Autodesk Fusion 360 part; units mm, degrees
(part 5 of 5)
  spline S33 degree 5 poles (-94.5307, 28.5823) (-94.5425, 28.575) (-94.566, 28.5604) (-94.6013, 28.5385) (-94.6482, 28.509) (-94.7065, 28.4721) (-94.7647, 28.4349) (-94.8226, 28.3975) (-94.8803, 28.3599) (-94.9377, 28.322) (-94.9949, 28.284) (-95.0518, 28.2458) (-95.1085, 28.2073) (-95.165, 28.1687) (-95.2212, 28.1298) (-95.2771, 28.0907) (-95.3328, 28.0514) (-95.3883, 28.0119) (-95.4435, 27.9721) (-95.4984, 27.9322) (-95.5531, 27.892) (-95.6074, 27.8517) (-95.6616, 27.8111) (-95.7154, 27.7703) (-95.769, 27.7293) (-95.8223, 27.688) (-95.8753, 27.6466) (-95.9281, 27.6049) (-95.9805, 27.563) (-96.0327, 27.5208) (-96.0845, 27.4785) (-96.1361, 27.4359) (-96.1874, 27.3931) (-96.2383, 27.3501) (-96.289, 27.3069) (-96.3393, 27.2634) (-96.3894, 27.2197) (-96.4391, 27.1758) (-96.4885, 27.1316) (-96.5375, 27.0872) (-96.5863, 27.0426) (-96.6346, 26.9977) (-96.6827, 26.9526) (-96.7303, 26.9073) (-96.7777, 26.8617) (-96.8246, 26.8158) (-96.8712, 26.7698) (-96.9175, 26.7234) (-96.9633, 26.6769) (-97.0088, 26.6301) (-97.0539, 26.583) (-97.0985, 26.5356) (-97.1427, 26.488) (-97.1865, 26.44) (-97.2298, 26.3918) (-97.2726, 26.3434) (-97.3151, 26.2946) (-97.3572, 26.2457) (-97.3988, 26.1965) (-97.44, 26.1469) (-97.4805, 26.0971) (-97.5204, 26.0468) (-97.5595, 25.9961) (-97.5979, 25.9449) (-97.6356, 25.8934) (-97.6728, 25.8417) (-97.7097, 25.7897) (-97.7462, 25.7375) (-97.7822, 25.6851) (-97.8172, 25.6321) (-97.8506, 25.5783) (-97.8756, 25.5344) (-97.8932, 25.5007) (-97.9043, 25.478) (-97.9097, 25.4666) knots -1 -1 -1 -1 -1 -1 -0.98571429 -0.97142857 -0.95714286 -0.94285714 -0.92857143 -0.91428571 -0.9 -0.88571429 -0.87142857 -0.85714286 -0.84285714 -0.82857143 -0.81428571 -0.8 -0.78571429 -0.77142857 -0.75714286 -0.74285714 -0.72857143 -0.71428571 -0.7 -0.68571429 -0.67142857 -0.65714286 -0.64285714 -0.62857143 -0.61428571 -0.6 -0.58571429 -0.57142857 -0.55714286 -0.54285714 -0.52857143 -0.51428571 -0.5 -0.48571429 -0.47142857 -0.45714286 -0.44285714 -0.42857143 -0.41428571 -0.4 -0.38571429 -0.37142857 -0.35714286 -0.34285714 -0.32857143 -0.31428571 -0.3 -0.28571429 -0.27142857 -0.25714286 -0.24285714 -0.22857143 -0.21428571 -0.2 -0.18571429 -0.17142857 -0.15714286 -0.14285714 -0.12857143 -0.11428571 -0.1 -0.08571429 -0.07142857 -0.05714286 -0.04285714 -0.02857143 -0.01428571 0 0 0 0 0 0
  line L33 (-97.9097, 25.4666) -> (-97.9531, 25.3753)
  arc A67 (-99.2529, 24.8861) -> (-97.9531, 25.3753) centre (-98.8565, 25.8041) ccw
  arc A68 (-99.2529, 24.8861) -> (-100.0022, 25.1964) centre (-110, 0) ccw
  arc A69 (-100.5754, 26.4615) -> (-100.0022, 25.1964) centre (-99.6334, 26.1259) ccw
  line L34 (-100.5754, 26.4615) -> (-100.5415, 26.5567)
  spline S34 degree 5 poles (-100.5415, 26.5567) (-100.5373, 26.5686) (-100.5291, 26.5926) (-100.5177, 26.6288) (-100.5043, 26.6775) (-100.4899, 26.7392) (-100.4772, 26.8014) (-100.4656, 26.8639) (-100.4545, 26.9266) (-100.4438, 26.9894) (-100.4335, 27.0524) (-100.4238, 27.1155) (-100.4148, 27.1788) (-100.4066, 27.2423) (-100.3992, 27.306) (-100.3926, 27.37) (-100.3867, 27.4341) (-100.3813, 27.4983) (-100.3765, 27.5627) (-100.372, 27.6272) (-100.3681, 27.6918) (-100.3646, 27.7565) (-100.3616, 27.8213) (-100.3592, 27.8862) (-100.3573, 27.9513) (-100.3559, 28.0164) (-100.3549, 28.0817) (-100.3544, 28.1471) (-100.3544, 28.2125) (-100.3547, 28.2781) (-100.3555, 28.3437) (-100.3568, 28.4094) (-100.3584, 28.4752) (-100.3605, 28.541) (-100.3629, 28.607) (-100.3658, 28.673) (-100.3691, 28.739) (-100.3728, 28.8052) (-100.3769, 28.8714) (-100.3814, 28.9377) (-100.3863, 29.004) (-100.3915, 29.0704) (-100.3971, 29.1369) (-100.4031, 29.2034) (-100.4095, 29.27) (-100.4162, 29.3366) (-100.4233, 29.4032) (-100.4308, 29.47) (-100.4386, 29.5367) (-100.4468, 29.6035) (-100.4553, 29.6704) (-100.4642, 29.7373) (-100.4734, 29.8042) (-100.483, 29.8712) (-100.4929, 29.9382) (-100.5031, 30.0052) (-100.5137, 30.0723) (-100.5247, 30.1394) (-100.5359, 30.2066) (-100.5475, 30.2738) (-100.5594, 30.341) (-100.5717, 30.4082) (-100.5843, 30.4755) (-100.5972, 30.5427) (-100.6104, 30.61) (-100.624, 30.6774) (-100.6378, 30.7447) (-100.652, 30.8121) (-100.6665, 30.8795) (-100.6813, 30.9469) (-100.6964, 31.0143) (-100.7088, 31.0683) (-100.7182, 31.1088) (-100.7245, 31.1357) (-100.7277, 31.1492) knots 0 0 0 0 0 0 0.01428571 0.02857143 0.04285714 0.05714286 0.07142857 0.08571429 0.1 0.11428571 0.12857143 0.14285714 0.15714286 0.17142857 0.18571429 0.2 0.21428571 0.22857143 0.24285714 0.25714286 0.27142857 0.28571429 0.3 0.31428571 0.32857143 0.34285714 0.35714286 0.37142857 0.38571429 0.4 0.41428571 0.42857143 0.44285714 0.45714286 0.47142857 0.48571429 0.5 0.51428571 0.52857143 0.54285714 0.55714286 0.57142857 0.58571429 0.6 0.61428571 0.62857143 0.64285714 0.65714286 0.67142857 0.68571429 0.7 0.71428571 0.72857143 0.74285714 0.75714286 0.77142857 0.78571429 0.8 0.81428571 0.82857143 0.84285714 0.85714286 0.87142857 0.88571429 0.9 0.91428571 0.92857143 0.94285714 0.95714286 0.97142857 0.98571429 1 1 1 1 1 1
  arc A70 (-100.7277, 31.1492) -> (-102.4554, 31.6122) centre (-110, 0) ccw
  spline S35 degree 5 poles (-102.4554, 31.6122) (-102.4649, 31.6021) (-102.4839, 31.5819) (-102.5123, 31.5515) (-102.55, 31.511) (-102.5968, 31.4601) (-102.6433, 31.4092) (-102.6896, 31.3581) (-102.7355, 31.3068) (-102.7812, 31.2554) (-102.8266, 31.2039) (-102.8717, 31.1522) (-102.9165, 31.1004) (-102.9611, 31.0484) (-103.0053, 30.9963) (-103.0492, 30.9441) (-103.0928, 30.8917) (-103.1362, 30.8392) (-103.1792, 30.7865) (-103.2219, 30.7337) (-103.2643, 30.6808) (-103.3064, 30.6277) (-103.3482, 30.5745) (-103.3896, 30.5212) (-103.4308, 30.4677) (-103.4716, 30.414) (-103.5121, 30.3603) (-103.5522, 30.3063) (-103.592, 30.2523) (-103.6315, 30.1981) (-103.6707, 30.1438) (-103.7094, 30.0893) (-103.7479, 30.0347) (-103.786, 29.98) (-103.8237, 29.9251) (-103.8611, 29.8701) (-103.8981, 29.8149) (-103.9348, 29.7596) (-103.971, 29.7042) (-104.0069, 29.6486) (-104.0425, 29.5929) (-104.0776, 29.537) (-104.1123, 29.481) (-104.1466, 29.4249) (-104.1805, 29.3686) (-104.214, 29.3121) (-104.2471, 29.2556) (-104.2798, 29.1989) (-104.312, 29.142) (-104.3439, 29.085) (-104.3752, 29.0279) (-104.4061, 28.9706) (-104.4364, 28.9131) (-104.4663, 28.8555) (-104.4956, 28.7977) (-104.5245, 28.7398) (-104.5529, 28.6818) (-104.5809, 28.6236) (-104.6083, 28.5653) (-104.6353, 28.5068) (-104.6615, 28.4481) (-104.687, 28.3892) (-104.7117, 28.3301) (-104.7355, 28.2708) (-104.7586, 28.2113) (-104.7812, 28.1516) (-104.8033, 28.0919) (-104.8251, 28.0321) (-104.8463, 27.9721) (-104.8664, 27.9119) (-104.8848, 27.8513) (-104.8975, 27.8023) (-104.9058, 27.7653) (-104.9107, 27.7405) (-104.9129, 27.728) knots -1 -1 -1 -1 -1 -1 -0.98571429 -0.97142857 -0.95714286 -0.94285714 -0.92857143 -0.91428571 -0.9 -0.88571429 -0.87142857 -0.85714286 -0.84285714 -0.82857143 -0.81428571 -0.8 -0.78571429 -0.77142857 -0.75714286 -0.74285714 -0.72857143 -0.71428571 -0.7 -0.68571429 -0.67142857 -0.65714286 -0.64285714 -0.62857143 -0.61428571 -0.6 -0.58571429 -0.57142857 -0.55714286 -0.54285714 -0.52857143 -0.51428571 -0.5 -0.48571429 -0.47142857 -0.45714286 -0.44285714 -0.42857143 -0.41428571 -0.4 -0.38571429 -0.37142857 -0.35714286 -0.34285714 -0.32857143 -0.31428571 -0.3 -0.28571429 -0.27142857 -0.25714286 -0.24285714 -0.22857143 -0.21428571 -0.2 -0.18571429 -0.17142857 -0.15714286 -0.14285714 -0.12857143 -0.11428571 -0.1 -0.08571429 -0.07142857 -0.05714286 -0.04285714 -0.02857143 -0.01428571 0 0 0 0 0 0
  line L35 (-104.9129, 27.728) -> (-104.9312, 27.6286)
  arc A71 (-106.0601, 26.8197) -> (-104.9312, 27.6286) centre (-105.9148, 27.809) ccw
  arc A72 (-106.0601, 26.8197) -> (-106.8642, 26.9255) centre (-110, 0) ccw
  arc A73 (-107.7453, 27.9991) -> (-106.8642, 26.9255) centre (-106.7485, 27.9188) ccw
  line L36 (-107.7453, 27.9991) -> (-107.7372, 28.0998)
  spline S36 degree 5 poles (-107.7372, 28.0998) (-107.7362, 28.1124) (-107.7345, 28.1377) (-107.7328, 28.1756) (-107.7325, 28.2262) (-107.7345, 28.2895) (-107.7384, 28.3528) (-107.7433, 28.4162) (-107.7489, 28.4797) (-107.7548, 28.5431) (-107.7612, 28.6066) (-107.7681, 28.67) (-107.7758, 28.7335) (-107.7843, 28.797) (-107.7937, 28.8605) (-107.8038, 28.9239) (-107.8147, 28.9874) (-107.8262, 29.0508) (-107.8381, 29.1143) (-107.8505, 29.1777) (-107.8634, 29.2411) (-107.8768, 29.3045) (-107.8907, 29.3679) (-107.9052, 29.4312) (-107.9202, 29.4946) (-107.9357, 29.5579) (-107.9516, 29.6212) (-107.9681, 29.6844) (-107.985, 29.7477) (-108.0023, 29.8109) (-108.02, 29.8741) (-108.0382, 29.9372) (-108.0568, 30.0003) (-108.0759, 30.0634) (-108.0953, 30.1264) (-108.1152, 30.1895) (-108.1355, 30.2524) (-108.1562, 30.3154) (-108.1773, 30.3783) (-108.1988, 30.4411) (-108.2206, 30.504) (-108.2429, 30.5667) (-108.2655, 30.6295) (-108.2885, 30.6922) (-108.3119, 30.7548) (-108.3356, 30.8174) (-108.3598, 30.88) (-108.3842, 30.9425) (-108.4091, 31.005) (-108.4342, 31.0674) (-108.4598, 31.1297) (-108.4857, 31.1921) (-108.5119, 31.2543) (-108.5385, 31.3165) (-108.5654, 31.3787) (-108.5927, 31.4408) (-108.6203, 31.5029) (-108.6482, 31.5649) (-108.6764, 31.6268) (-108.705, 31.6887) (-108.7339, 31.7505) (-108.7632, 31.8123) (-108.7927, 31.874) (-108.8226, 31.9356) (-108.8528, 31.9972) (-108.8833, 32.0588) (-108.9142, 32.1202) (-108.9453, 32.1816) (-108.9767, 32.243) (-109.0085, 32.3043) (-109.0406, 32.3655) (-109.0664, 32.4144) (-109.086, 32.4511) (-109.0991, 32.4755) (-109.1057, 32.4877) knots 0 0 0 0 0 0 0.01428571 0.02857143 0.04285714 0.05714286 0.07142857 0.08571429 0.1 0.11428571 0.12857143 0.14285714 0.15714286 0.17142857 0.18571429 0.2 0.21428571 0.22857143 0.24285714 0.25714286 0.27142857 0.28571429 0.3 0.31428571 0.32857143 0.34285714 0.35714286 0.37142857 0.38571429 0.4 0.41428571 0.42857143 0.44285714 0.45714286 0.47142857 0.48571429 0.5 0.51428571 0.52857143 0.54285714 0.55714286 0.57142857 0.58571429 0.6 0.61428571 0.62857143 0.64285714 0.65714286 0.67142857 0.68571429 0.7 0.71428571 0.72857143 0.74285714 0.75714286 0.77142857 0.78571429 0.8 0.81428571 0.82857143 0.84285714 0.85714286 0.87142857 0.88571429 0.9 0.91428571 0.92857143 0.94285714 0.95714286 0.97142857 0.98571429 1 1 1 1 1 1
  arc A74 (-109.1057, 32.4877) -> (-110.8943, 32.4877) centre (-110, 0) ccw
  spline S37 degree 5 poles (-110.8943, 32.4877) (-110.9009, 32.4755) (-110.914, 32.4511) (-110.9336, 32.4144) (-110.9594, 32.3655) (-110.9915, 32.3043) (-111.0233, 32.243) (-111.0547, 32.1816) (-111.0858, 32.1202) (-111.1167, 32.0588) (-111.1472, 31.9972) (-111.1774, 31.9356) (-111.2073, 31.874) (-111.2368, 31.8123) (-111.2661, 31.7505) (-111.295, 31.6887) (-111.3236, 31.6268) (-111.3518, 31.5649) (-111.3797, 31.5029) (-111.4073, 31.4408) (-111.4346, 31.3787) (-111.4615, 31.3165) (-111.4881, 31.2543) (-111.5143, 31.1921) (-111.5402, 31.1297) (-111.5658, 31.0674) (-111.5909, 31.005) (-111.6158, 30.9425) (-111.6402, 30.88) (-111.6644, 30.8174) (-111.6881, 30.7548) (-111.7115, 30.6922) (-111.7345, 30.6295) (-111.7571, 30.5667) (-111.7794, 30.504) (-111.8012, 30.4411) (-111.8227, 30.3783) (-111.8438, 30.3154) (-111.8645, 30.2524) (-111.8848, 30.1895) (-111.9047, 30.1264) (-111.9241, 30.0634) (-111.9432, 30.0003) (-111.9618, 29.9372) (-111.98, 29.8741) (-111.9977, 29.8109) (-112.015, 29.7477) (-112.0319, 29.6844) (-112.0484, 29.6212) (-112.0643, 29.5579) (-112.0798, 29.4946) (-112.0948, 29.4312) (-112.1093, 29.3679) (-112.1232, 29.3045) (-112.1366, 29.2411) (-112.1495, 29.1777) (-112.1619, 29.1143) (-112.1738, 29.0508) (-112.1853, 28.9874) (-112.1962, 28.9239) (-112.2063, 28.8605) (-112.2157, 28.797) (-112.2242, 28.7335) (-112.2319, 28.67) (-112.2388, 28.6066) (-112.2452, 28.5431) (-112.2511, 28.4797) (-112.2567, 28.4162) (-112.2616, 28.3528) (-112.2655, 28.2895) (-112.2675, 28.2262) (-112.2672, 28.1756) (-112.2655, 28.1377) (-112.2638, 28.1124) (-112.2628, 28.0998) knots -1 -1 -1 -1 -1 -1 -0.98571429 -0.97142857 -0.95714286 -0.94285714 -0.92857143 -0.91428571 -0.9 -0.88571429 -0.87142857 -0.85714286 -0.84285714 -0.82857143 -0.81428571 -0.8 -0.78571429 -0.77142857 -0.75714286 -0.74285714 -0.72857143 -0.71428571 -0.7 -0.68571429 -0.67142857 -0.65714286 -0.64285714 -0.62857143 -0.61428571 -0.6 -0.58571429 -0.57142857 -0.55714286 -0.54285714 -0.52857143 -0.51428571 -0.5 -0.48571429 -0.47142857 -0.45714286 -0.44285714 -0.42857143 -0.41428571 -0.4 -0.38571429 -0.37142857 -0.35714286 -0.34285714 -0.32857143 -0.31428571 -0.3 -0.28571429 -0.27142857 -0.25714286 -0.24285714 -0.22857143 -0.21428571 -0.2 -0.18571429 -0.17142857 -0.15714286 -0.14285714 -0.12857143 -0.11428571 -0.1 -0.08571429 -0.07142857 -0.05714286 -0.04285714 -0.02857143 -0.01428571 0 0 0 0 0 0
  line L37 (-112.2628, 28.0998) -> (-112.2547, 27.9991)
  arc A75 (-113.1358, 26.9255) -> (-112.2547, 27.9991) centre (-113.2515, 27.9188) ccw
  arc A76 (-113.1358, 26.9255) -> (-113.9399, 26.8197) centre (-110, 0) ccw
  arc A77 (-115.0688, 27.6286) -> (-113.9399, 26.8197) centre (-114.0852, 27.809) ccw
  line L38 (-115.0688, 27.6286) -> (-115.0871, 27.728)
  spline S38 degree 5 poles (-115.0871, 27.728) (-115.0893, 27.7405) (-115.0942, 27.7653) (-115.1025, 27.8023) (-115.1152, 27.8513) (-115.1336, 27.9119) (-115.1537, 27.9721) (-115.1749, 28.0321) (-115.1967, 28.0919) (-115.2188, 28.1516) (-115.2414, 28.2113) (-115.2645, 28.2708) (-115.2883, 28.3301) (-115.313, 28.3892) (-115.3385, 28.4481) (-115.3647, 28.5068) (-115.3917, 28.5653) (-115.4191, 28.6236) (-115.4471, 28.6818) (-115.4755, 28.7398) (-115.5044, 28.7977) (-115.5337, 28.8555) (-115.5636, 28.9131) (-115.5939, 28.9706) (-115.6248, 29.0279) (-115.6561, 29.085) (-115.688, 29.142) (-115.7202, 29.1989) (-115.7529, 29.2556) (-115.786, 29.3121) (-115.8195, 29.3686) (-115.8534, 29.4249) (-115.8877, 29.481) (-115.9224, 29.537) (-115.9575, 29.5929) (-115.9931, 29.6486) (-116.029, 29.7042) (-116.0652, 29.7596) (-116.1019, 29.8149) (-116.1389, 29.8701) (-116.1763, 29.9251) (-116.214, 29.98) (-116.2521, 30.0347) (-116.2906, 30.0893) (-116.3293, 30.1438) (-116.3685, 30.1981) (-116.408, 30.2523) (-116.4478, 30.3063) (-116.4879, 30.3603) (-116.5284, 30.414) (-116.5692, 30.4677) (-116.6104, 30.5212) (-116.6518, 30.5745) (-116.6936, 30.6277) (-116.7357, 30.6808) (-116.7781, 30.7337) (-116.8208, 30.7865) (-116.8638, 30.8392) (-116.9072, 30.8917) (-116.9508, 30.9441) (-116.9947, 30.9963) (-117.0389, 31.0484) (-117.0835, 31.1004) (-117.1283, 31.1522) (-117.1734, 31.2039) (-117.2188, 31.2554) (-117.2645, 31.3068) (-117.3104, 31.3581) (-117.3567, 31.4092) (-117.4032, 31.4601) (-117.45, 31.511) (-117.4877, 31.5515) (-117.5161, 31.5819) (-117.5351, 31.6021) (-117.5446, 31.6122) knots 0 0 0 0 0 0 0.01428571 0.02857143 0.04285714 0.05714286 0.07142857 0.08571429 0.1 0.11428571 0.12857143 0.14285714 0.15714286 0.17142857 0.18571429 0.2 0.21428571 0.22857143 0.24285714 0.25714286 0.27142857 0.28571429 0.3 0.31428571 0.32857143 0.34285714 0.35714286 0.37142857 0.38571429 0.4 0.41428571 0.42857143 0.44285714 0.45714286 0.47142857 0.48571429 0.5 0.51428571 0.52857143 0.54285714 0.55714286 0.57142857 0.58571429 0.6 0.61428571 0.62857143 0.64285714 0.65714286 0.67142857 0.68571429 0.7 0.71428571 0.72857143 0.74285714 0.75714286 0.77142857 0.78571429 0.8 0.81428571 0.82857143 0.84285714 0.85714286 0.87142857 0.88571429 0.9 0.91428571 0.92857143 0.94285714 0.95714286 0.97142857 0.98571429 1 1 1 1 1 1
  arc A78 (-117.5446, 31.6122) -> (-119.2723, 31.1492) centre (-110, 0) ccw
  spline S39 degree 5 poles (-119.2723, 31.1492) (-119.2755, 31.1357) (-119.2818, 31.1088) (-119.2912, 31.0683) (-119.3036, 31.0143) (-119.3187, 30.9469) (-119.3335, 30.8795) (-119.348, 30.8121) (-119.3622, 30.7447) (-119.376, 30.6774) (-119.3896, 30.61) (-119.4028, 30.5427) (-119.4157, 30.4755) (-119.4283, 30.4082) (-119.4406, 30.341) (-119.4525, 30.2738) (-119.4641, 30.2066) (-119.4753, 30.1394) (-119.4863, 30.0723) (-119.4969, 30.0052) (-119.5071, 29.9382) (-119.517, 29.8712) (-119.5266, 29.8042) (-119.5358, 29.7373) (-119.5447, 29.6704) (-119.5532, 29.6035) (-119.5614, 29.5367) (-119.5692, 29.47) (-119.5767, 29.4032) (-119.5838, 29.3366) (-119.5905, 29.27) (-119.5969, 29.2034) (-119.6029, 29.1369) (-119.6085, 29.0704) (-119.6137, 29.004) (-119.6186, 28.9377) (-119.6231, 28.8714) (-119.6272, 28.8052) (-119.6309, 28.739) (-119.6342, 28.673) (-119.6371, 28.607) (-119.6395, 28.541) (-119.6416, 28.4752) (-119.6432, 28.4094) (-119.6445, 28.3437) (-119.6453, 28.2781) (-119.6456, 28.2125) (-119.6456, 28.1471) (-119.6451, 28.0817) (-119.6441, 28.0164) (-119.6427, 27.9513) (-119.6408, 27.8862) (-119.6384, 27.8213) (-119.6354, 27.7565) (-119.6319, 27.6918) (-119.628, 27.6272) (-119.6235, 27.5627) (-119.6187, 27.4983) (-119.6133, 27.4341) (-119.6074, 27.37) (-119.6008, 27.306) (-119.5934, 27.2423) (-119.5852, 27.1788) (-119.5762, 27.1155) (-119.5665, 27.0524) (-119.5562, 26.9894) (-119.5455, 26.9266) (-119.5344, 26.8639) (-119.5228, 26.8014) (-119.5101, 26.7392) (-119.4957, 26.6775) (-119.4823, 26.6288) (-119.4709, 26.5926) (-119.4627, 26.5686) (-119.4585, 26.5567) knots -1 -1 -1 -1 -1 -1 -0.98571429 -0.97142857 -0.95714286 -0.94285714 -0.92857143 -0.91428571 -0.9 -0.88571429 -0.87142857 -0.85714286 -0.84285714 -0.82857143 -0.81428571 -0.8 -0.78571429 -0.77142857 -0.75714286 -0.74285714 -0.72857143 -0.71428571 -0.7 -0.68571429 -0.67142857 -0.65714286 -0.64285714 -0.62857143 -0.61428571 -0.6 -0.58571429 -0.57142857 -0.55714286 -0.54285714 -0.52857143 -0.51428571 -0.5 -0.48571429 -0.47142857 -0.45714286 -0.44285714 -0.42857143 -0.41428571 -0.4 -0.38571429 -0.37142857 -0.35714286 -0.34285714 -0.32857143 -0.31428571 -0.3 -0.28571429 -0.27142857 -0.25714286 -0.24285714 -0.22857143 -0.21428571 -0.2 -0.18571429 -0.17142857 -0.15714286 -0.14285714 -0.12857143 -0.11428571 -0.1 -0.08571429 -0.07142857 -0.05714286 -0.04285714 -0.02857143 -0.01428571 0 0 0 0 0 0
  line L39 (-119.4585, 26.5567) -> (-119.4246, 26.4615)
  arc A79 (-119.9978, 25.1964) -> (-119.4246, 26.4615) centre (-120.3666, 26.1259) ccw
  arc A80 (-119.9978, 25.1964) -> (-120.7471, 24.8861) centre (-110, 0) ccw
  arc A81 (-122.0469, 25.3753) -> (-120.7471, 24.8861) centre (-121.1435, 25.8041) ccw
  line L40 (-122.0469, 25.3753) -> (-122.0903, 25.4666)
  spline S40 degree 5 poles (-122.0903, 25.4666) (-122.0957, 25.478) (-122.1068, 25.5007) (-122.1244, 25.5344) (-122.1494, 25.5783) (-122.1828, 25.6321) (-122.2178, 25.6851) (-122.2538, 25.7375) (-122.2903, 25.7897) (-122.3272, 25.8417) (-122.3644, 25.8934) (-122.4021, 25.9449) (-122.4405, 25.9961) (-122.4796, 26.0468) (-122.5195, 26.0971) (-122.56, 26.1469) (-122.6012, 26.1965) (-122.6428, 26.2457) (-122.6849, 26.2946) (-122.7274, 26.3434) (-122.7702, 26.3918) (-122.8135, 26.44) (-122.8573, 26.488) (-122.9015, 26.5356) (-122.9461, 26.583) (-122.9912, 26.6301) (-123.0367, 26.6769) (-123.0825, 26.7234) (-123.1288, 26.7698) (-123.1754, 26.8158) (-123.2223, 26.8617) (-123.2697, 26.9073) (-123.3173, 26.9526) (-123.3654, 26.9977) (-123.4137, 27.0426) (-123.4625, 27.0872) (-123.5115, 27.1316) (-123.5609, 27.1758) (-123.6106, 27.2197) (-123.6607, 27.2634) (-123.711, 27.3069) (-123.7617, 27.3501) (-123.8126, 27.3931) (-123.8639, 27.4359) (-123.9155, 27.4785) (-123.9673, 27.5208) (-124.0195, 27.563) (-124.0719, 27.6049) (-124.1247, 27.6466) (-124.1777, 27.688) (-124.231, 27.7293) (-124.2846, 27.7703) (-124.3384, 27.8111) (-124.3926, 27.8517) (-124.4469, 27.892) (-124.5016, 27.9322) (-124.5565, 27.9721) (-124.6117, 28.0119) (-124.6672, 28.0514) (-124.7229, 28.0907) (-124.7788, 28.1298) (-124.835, 28.1687) (-124.8915, 28.2073) (-124.9482, 28.2458) (-125.0051, 28.284) (-125.0623, 28.322) (-125.1197, 28.3599) (-125.1774, 28.3975) (-125.2353, 28.4349) (-125.2935, 28.4721) (-125.3518, 28.509) (-125.3987, 28.5385) (-125.434, 28.5604) (-125.4575, 28.575) (-125.4693, 28.5823) knots 0 0 0 0 0 0 0.01428571 0.02857143 0.04285714 0.05714286 0.07142857 0.08571429 0.1 0.11428571 0.12857143 0.14285714 0.15714286 0.17142857 0.18571429 0.2 0.21428571 0.22857143 0.24285714 0.25714286 0.27142857 0.28571429 0.3 0.31428571 0.32857143 0.34285714 0.35714286 0.37142857 0.38571429 0.4 0.41428571 0.42857143 0.44285714 0.45714286 0.47142857 0.48571429 0.5 0.51428571 0.52857143 0.54285714 0.55714286 0.57142857 0.58571429 0.6 0.61428571 0.62857143 0.64285714 0.65714286 0.67142857 0.68571429 0.7 0.71428571 0.72857143 0.74285714 0.75714286 0.77142857 0.78571429 0.8 0.81428571 0.82857143 0.84285714 0.85714286 0.87142857 0.88571429 0.9 0.91428571 0.92857143 0.94285714 0.95714286 0.97142857 0.98571429 1 1 1 1 1 1
  arc A82 (-125.4693, 28.5823) -> (-127.0184, 27.688) centre (-110, 0) ccw
  spline S41 degree 5 poles (-127.0184, 27.688) (-127.0179, 27.6741) (-127.0171, 27.6464) (-127.0157, 27.6049) (-127.0136, 27.5496) (-127.0108, 27.4806) (-127.0077, 27.4116) (-127.0042, 27.3428) (-127.0005, 27.274) (-126.9965, 27.2054) (-126.9921, 27.1368) (-126.9875, 27.0684) (-126.9825, 27.0001) (-126.9773, 26.9318) (-126.9717, 26.8637) (-126.9658, 26.7957) (-126.9596, 26.7278) (-126.9531, 26.6601) (-126.9463, 26.5924) (-126.9392, 26.5249) (-126.9317, 26.4574) (-126.924, 26.3902) (-126.9159, 26.323) (-126.9075, 26.2559) (-126.8987, 26.189) (-126.8897, 26.1223) (-126.8803, 26.0556) (-126.8705, 25.9891) (-126.8605, 25.9227) (-126.8501, 25.8565) (-126.8393, 25.7904) (-126.8283, 25.7245) (-126.8168, 25.6587) (-126.8051, 25.593) (-126.7929, 25.5275) (-126.7805, 25.4622) (-126.7676, 25.397) (-126.7545, 25.332) (-126.7409, 25.2671) (-126.727, 25.2025) (-126.7127, 25.1379) (-126.698, 25.0736) (-126.683, 25.0095) (-126.6676, 24.9455) (-126.6517, 24.8817) (-126.6355, 24.8181) (-126.6189, 24.7547) (-126.6019, 24.6915) (-126.5845, 24.6285) (-126.5667, 24.5657) (-126.5485, 24.5031) (-126.5298, 24.4408) (-126.5106, 24.3787) (-126.491, 24.3169) (-126.4709, 24.2553) (-126.4503, 24.1939) (-126.4294, 24.1328) (-126.408, 24.0718) (-126.3862, 24.0112) (-126.3639, 23.9508) (-126.341, 23.8907) (-126.3174, 23.8311) (-126.293, 23.7718) (-126.2679, 23.713) (-126.2422, 23.6546) (-126.2159, 23.5965) (-126.1894, 23.5386) (-126.1625, 23.4809) (-126.135, 23.4235) (-126.1067, 23.3667) (-126.0768, 23.3108) (-126.0512, 23.2672) (-126.0309, 23.2352) (-126.0168, 23.2142) (-126.0096, 23.2037) knots -1 -1 -1 -1 -1 -1 -0.98571429 -0.97142857 -0.95714286 -0.94285714 -0.92857143 -0.91428571 -0.9 -0.88571429 -0.87142857 -0.85714286 -0.84285714 -0.82857143 -0.81428571 -0.8 -0.78571429 -0.77142857 -0.75714286 -0.74285714 -0.72857143 -0.71428571 -0.7 -0.68571429 -0.67142857 -0.65714286 -0.64285714 -0.62857143 -0.61428571 -0.6 -0.58571429 -0.57142857 -0.55714286 -0.54285714 -0.52857143 -0.51428571 -0.5 -0.48571429 -0.47142857 -0.45714286 -0.44285714 -0.42857143 -0.41428571 -0.4 -0.38571429 -0.37142857 -0.35714286 -0.34285714 -0.32857143 -0.31428571 -0.3 -0.28571429 -0.27142857 -0.25714286 -0.24285714 -0.22857143 -0.21428571 -0.2 -0.18571429 -0.17142857 -0.15714286 -0.14285714 -0.12857143 -0.11428571 -0.1 -0.08571429 -0.07142857 -0.05714286 -0.04285714 -0.02857143 -0.01428571 0 0 0 0 0 0
  line L41 (-126.0096, 23.2037) -> (-125.9522, 23.1206)
  arc A83 (-126.1784, 21.7503) -> (-125.9522, 23.1206) centre (-126.7753, 22.5527) ccw
  arc A84 (-126.1784, 21.7503) -> (-126.8219, 21.2566) centre (-110, 0) ccw
  arc A85 (-128.204, 21.3926) -> (-126.8219, 21.2566) centre (-127.4424, 22.0407) ccw
  line L42 (-128.204, 21.3926) -> (-128.2695, 21.4696)
  spline S42 degree 5 poles (-128.2695, 21.4696) (-128.2777, 21.4793) (-128.2944, 21.4983) (-128.32, 21.5263) (-128.3556, 21.5623) (-128.4018, 21.6056) (-128.4493, 21.6477) (-128.4976, 21.689) (-128.5464, 21.73) (-128.5954, 21.7706) (-128.6448, 21.811) (-128.6946, 21.851) (-128.7449, 21.8904) (-128.7958, 21.9293) (-128.8473, 21.9675) (-128.8994, 22.0052) (-128.9519, 22.0424) (-129.0049, 22.0792) (-129.0582, 22.1156) (-129.1119, 22.1516) (-129.1658, 22.1874) (-129.2201, 22.2227) (-129.2748, 22.2577) (-129.3298, 22.2923) (-129.3852, 22.3265) (-129.4409, 22.3603) (-129.4969, 22.3937) (-129.5533, 22.4268) (-129.6099, 22.4596) (-129.6669, 22.4921) (-129.7241, 22.5242) (-129.7816, 22.556) (-129.8394, 22.5875) (-129.8975, 22.6186) (-129.9558, 22.6494) (-130.0144, 22.6799) (-130.0733, 22.7101) (-130.1325, 22.74) (-130.1918, 22.7695) (-130.2515, 22.7988) (-130.3114, 22.8277) (-130.3715, 22.8564) (-130.4318, 22.8848) (-130.4924, 22.9128) (-130.5533, 22.9406) (-130.6143, 22.9681) (-130.6756, 22.9953) (-130.7371, 23.0222) (-130.7988, 23.0488) (-130.8608, 23.0751) (-130.923, 23.1011) (-130.9853, 23.1269) (-131.0479, 23.1524) (-131.1107, 23.1776) (-131.1737, 23.2025) (-131.2369, 23.2271) (-131.3003, 23.2515) (-131.3638, 23.2756) (-131.4276, 23.2994) (-131.4916, 23.323) (-131.5558, 23.3462) (-131.6201, 23.3693) (-131.6847, 23.392) (-131.7494, 23.4145) (-131.8143, 23.4367) (-131.8794, 23.4586) (-131.9446, 23.4803) (-132.0101, 23.5017) (-132.0757, 23.5228) (-132.1415, 23.5437) (-132.2074, 23.5643) (-132.2603, 23.5806) (-132.3001, 23.5927) (-132.3266, 23.6007) (-132.3399, 23.6047) knots 0 0 0 0 0 0 0.01428571 0.02857143 0.04285714 0.05714286 0.07142857 0.08571429 0.1 0.11428571 0.12857143 0.14285714 0.15714286 0.17142857 0.18571429 0.2 0.21428571 0.22857143 0.24285714 0.25714286 0.27142857 0.28571429 0.3 0.31428571 0.32857143 0.34285714 0.35714286 0.37142857 0.38571429 0.4 0.41428571 0.42857143 0.44285714 0.45714286 0.47142857 0.48571429 0.5 0.51428571 0.52857143 0.54285714 0.55714286 0.57142857 0.58571429 0.6 0.61428571 0.62857143 0.64285714 0.65714286 0.67142857 0.68571429 0.7 0.71428571 0.72857143 0.74285714 0.75714286 0.77142857 0.78571429 0.8 0.81428571 0.82857143 0.84285714 0.85714286 0.87142857 0.88571429 0.9 0.91428571 0.92857143 0.94285714 0.95714286 0.97142857 0.98571429 1 1 1 1 1 1
  arc A86 (-132.3399, 23.6047) -> (-133.6047, 22.3399) centre (-110, 0) ccw
  spline S43 degree 5 poles (-133.6047, 22.3399) (-133.6007, 22.3266) (-133.5927, 22.3001) (-133.5806, 22.2603) (-133.5643, 22.2074) (-133.5437, 22.1415) (-133.5228, 22.0757) (-133.5017, 22.0101) (-133.4803, 21.9446) (-133.4586, 21.8794) (-133.4367, 21.8143) (-133.4145, 21.7494) (-133.392, 21.6847) (-133.3693, 21.6201) (-133.3462, 21.5558) (-133.323, 21.4916) (-133.2994, 21.4276) (-133.2756, 21.3638) (-133.2515, 21.3003) (-133.2271, 21.2369) (-133.2025, 21.1737) (-133.1776, 21.1107) (-133.1524, 21.0479) (-133.1269, 20.9853) (-133.1011, 20.923) (-133.0751, 20.8608) (-133.0488, 20.7988) (-133.0222, 20.7371) (-132.9953, 20.6756) (-132.9681, 20.6143) (-132.9406, 20.5533) (-132.9128, 20.4924) (-132.8848, 20.4318) (-132.8564, 20.3715) (-132.8277, 20.3114) (-132.7988, 20.2515) (-132.7695, 20.1918) (-132.74, 20.1325) (-132.7101, 20.0733) (-132.6799, 20.0144) (-132.6494, 19.9558) (-132.6186, 19.8975) (-132.5875, 19.8394) (-132.556, 19.7816) (-132.5242, 19.7241) (-132.4921, 19.6669) (-132.4596, 19.6099) (-132.4268, 19.5533) (-132.3937, 19.4969) (-132.3603, 19.4409) (-132.3265, 19.3852) (-132.2923, 19.3298) (-132.2577, 19.2748) (-132.2227, 19.2201) (-132.1874, 19.1658) (-132.1516, 19.1119) (-132.1156, 19.0582) (-132.0792, 19.0049) (-132.0424, 18.9519) (-132.0052, 18.8994) (-131.9675, 18.8473) (-131.9293, 18.7958) (-131.8904, 18.7449) (-131.851, 18.6946) (-131.811, 18.6448) (-131.7706, 18.5954) (-131.73, 18.5464) (-131.689, 18.4976) (-131.6477, 18.4493) (-131.6056, 18.4018) (-131.5623, 18.3556) (-131.5263, 18.32) (-131.4983, 18.2944) (-131.4793, 18.2777) (-131.4696, 18.2695) knots -1 -1 -1 -1 -1 -1 -0.98571429 -0.97142857 -0.95714286 -0.94285714 -0.92857143 -0.91428571 -0.9 -0.88571429 -0.87142857 -0.85714286 -0.84285714 -0.82857143 -0.81428571 -0.8 -0.78571429 -0.77142857 -0.75714286 -0.74285714 -0.72857143 -0.71428571 -0.7 -0.68571429 -0.67142857 -0.65714286 -0.64285714 -0.62857143 -0.61428571 -0.6 -0.58571429 -0.57142857 -0.55714286 -0.54285714 -0.52857143 -0.51428571 -0.5 -0.48571429 -0.47142857 -0.45714286 -0.44285714 -0.42857143 -0.41428571 -0.4 -0.38571429 -0.37142857 -0.35714286 -0.34285714 -0.32857143 -0.31428571 -0.3 -0.28571429 -0.27142857 -0.25714286 -0.24285714 -0.22857143 -0.21428571 -0.2 -0.18571429 -0.17142857 -0.15714286 -0.14285714 -0.12857143 -0.11428571 -0.1 -0.08571429 -0.07142857 -0.05714286 -0.04285714 -0.02857143 -0.01428571 0 0 0 0 0 0
  line L43 (-131.4696, 18.2695) -> (-131.3926, 18.204)
  arc A87 (-131.2566, 16.8219) -> (-131.3926, 18.204) centre (-132.0407, 17.4424) ccw
  arc A88 (-131.2566, 16.8219) -> (-131.7503, 16.1784) centre (-110, 0) ccw
  arc A89 (-133.1206, 15.9522) -> (-131.7503, 16.1784) centre (-132.5527, 16.7753) ccw
  line L44 (-133.1206, 15.9522) -> (-133.2037, 16.0096)
  spline S44 degree 5 poles (-133.2037, 16.0096) (-133.2142, 16.0168) (-133.2352, 16.0309) (-133.2672, 16.0512) (-133.3108, 16.0768) (-133.3667, 16.1067) (-133.4235, 16.135) (-133.4809, 16.1625) (-133.5386, 16.1894) (-133.5965, 16.2159) (-133.6546, 16.2422) (-133.713, 16.2679) (-133.7718, 16.293) (-133.8311, 16.3174) (-133.8907, 16.341) (-133.9508, 16.3639) (-134.0112, 16.3862) (-134.0718, 16.408) (-134.1328, 16.4294) (-134.1939, 16.4503) (-134.2553, 16.4709) (-134.3169, 16.491) (-134.3787, 16.5106) (-134.4408, 16.5298) (-134.5031, 16.5485) (-134.5657, 16.5667) (-134.6285, 16.5845) (-134.6915, 16.6019) (-134.7547, 16.6189) (-134.8181, 16.6355) (-134.8817, 16.6517) (-134.9455, 16.6676) (-135.0095, 16.683) (-135.0736, 16.698) (-135.1379, 16.7127) (-135.2025, 16.727) (-135.2671, 16.7409) (-135.332, 16.7545) (-135.397, 16.7676) (-135.4622, 16.7805) (-135.5275, 16.7929) (-135.593, 16.8051) (-135.6587, 16.8168) (-135.7245, 16.8283) (-135.7904, 16.8393) (-135.8565, 16.8501) (-135.9227, 16.8605) (-135.9891, 16.8705) (-136.0556, 16.8803) (-136.1223, 16.8897) (-136.189, 16.8987) (-136.2559, 16.9075) (-136.323, 16.9159) (-136.3902, 16.924) (-136.4574, 16.9317) (-136.5249, 16.9392) (-136.5924, 16.9463) (-136.6601, 16.9531) (-136.7278, 16.9596) (-136.7957, 16.9658) (-136.8637, 16.9717) (-136.9318, 16.9773) (-137.0001, 16.9825) (-137.0684, 16.9875) (-137.1368, 16.9921) (-137.2054, 16.9965) (-137.274, 17.0005) (-137.3428, 17.0042) (-137.4116, 17.0077) (-137.4806, 17.0108) (-137.5496, 17.0136) (-137.6049, 17.0157) (-137.6464, 17.0171) (-137.6741, 17.0179) (-137.688, 17.0184) knots 0 0 0 0 0 0 0.01428571 0.02857143 0.04285714 0.05714286 0.07142857 0.08571429 0.1 0.11428571 0.12857143 0.14285714 0.15714286 0.17142857 0.18571429 0.2 0.21428571 0.22857143 0.24285714 0.25714286 0.27142857 0.28571429 0.3 0.31428571 0.32857143 0.34285714 0.35714286 0.37142857 0.38571429 0.4 0.41428571 0.42857143 0.44285714 0.45714286 0.47142857 0.48571429 0.5 0.51428571 0.52857143 0.54285714 0.55714286 0.57142857 0.58571429 0.6 0.61428571 0.62857143 0.64285714 0.65714286 0.67142857 0.68571429 0.7 0.71428571 0.72857143 0.74285714 0.75714286 0.77142857 0.78571429 0.8 0.81428571 0.82857143 0.84285714 0.85714286 0.87142857 0.88571429 0.9 0.91428571 0.92857143 0.94285714 0.95714286 0.97142857 0.98571429 1 1 1 1 1 1
  arc A90 (-137.688, 17.0184) -> (-138.5823, 15.4693) centre (-110, 0) ccw
  spline S45 degree 5 poles (-138.5823, 15.4693) (-138.575, 15.4575) (-138.5604, 15.434) (-138.5385, 15.3987) (-138.509, 15.3518) (-138.4721, 15.2935) (-138.4349, 15.2353) (-138.3975, 15.1774) (-138.3599, 15.1197) (-138.322, 15.0623) (-138.284, 15.0051) (-138.2458, 14.9482) (-138.2073, 14.8915) (-138.1687, 14.835) (-138.1298, 14.7788) (-138.0907, 14.7229) (-138.0514, 14.6672) (-138.0119, 14.6117) (-137.9721, 14.5565) (-137.9322, 14.5016) (-137.892, 14.4469) (-137.8517, 14.3926) (-137.8111, 14.3384) (-137.7703, 14.2846) (-137.7293, 14.231) (-137.688, 14.1777) (-137.6466, 14.1247) (-137.6049, 14.0719) (-137.563, 14.0195) (-137.5208, 13.9673) (-137.4785, 13.9155) (-137.4359, 13.8639) (-137.3931, 13.8126) (-137.3501, 13.7617) (-137.3069, 13.711) (-137.2634, 13.6607) (-137.2197, 13.6106) (-137.1758, 13.5609) (-137.1316, 13.5115) (-137.0872, 13.4625) (-137.0426, 13.4137) (-136.9977, 13.3654) (-136.9526, 13.3173) (-136.9073, 13.2697) (-136.8617, 13.2223) (-136.8158, 13.1754) (-136.7698, 13.1288) (-136.7234, 13.0825) (-136.6769, 13.0367) (-136.6301, 12.9912) (-136.583, 12.9461) (-136.5356, 12.9015) (-136.488, 12.8573) (-136.44, 12.8135) (-136.3918, 12.7702) (-136.3434, 12.7274) (-136.2946, 12.6849) (-136.2457, 12.6428) (-136.1965, 12.6012) (-136.1469, 12.56) (-136.0971, 12.5195) (-136.0468, 12.4796) (-135.9961, 12.4405) (-135.9449, 12.4021) (-135.8934, 12.3644) (-135.8417, 12.3272) (-135.7897, 12.2903) (-135.7375, 12.2538) (-135.6851, 12.2178) (-135.6321, 12.1828) (-135.5783, 12.1494) (-135.5344, 12.1244) (-135.5007, 12.1068) (-135.478, 12.0957) (-135.4666, 12.0903) knots -1 -1 -1 -1 -1 -1 -0.98571429 -0.97142857 -0.95714286 -0.94285714 -0.92857143 -0.91428571 -0.9 -0.88571429 -0.87142857 -0.85714286 -0.84285714 -0.82857143 -0.81428571 -0.8 -0.78571429 -0.77142857 -0.75714286 -0.74285714 -0.72857143 -0.71428571 -0.7 -0.68571429 -0.67142857 -0.65714286 -0.64285714 -0.62857143 -0.61428571 -0.6 -0.58571429 -0.57142857 -0.55714286 -0.54285714 -0.52857143 -0.51428571 -0.5 -0.48571429 -0.47142857 -0.45714286 -0.44285714 -0.42857143 -0.41428571 -0.4 -0.38571429 -0.37142857 -0.35714286 -0.34285714 -0.32857143 -0.31428571 -0.3 -0.28571429 -0.27142857 -0.25714286 -0.24285714 -0.22857143 -0.21428571 -0.2 -0.18571429 -0.17142857 -0.15714286 -0.14285714 -0.12857143 -0.11428571 -0.1 -0.08571429 -0.07142857 -0.05714286 -0.04285714 -0.02857143 -0.01428571 0 0 0 0 0 0
  line L45 (-135.4666, 12.0903) -> (-135.3753, 12.0469)
  arc A91 (-134.8861, 10.7471) -> (-135.3753, 12.0469) centre (-135.8041, 11.1435) ccw
  arc A92 (-134.8861, 10.7471) -> (-135.1964, 9.9978) centre (-110, 0) ccw
  arc A93 (-136.4615, 9.4246) -> (-135.1964, 9.9978) centre (-136.1259, 10.3666) ccw
  line L46 (-136.4615, 9.4246) -> (-136.5567, 9.4585)
  spline S46 degree 5 poles (-136.5567, 9.4585) (-136.5686, 9.4627) (-136.5926, 9.4709) (-136.6288, 9.4823) (-136.6775, 9.4957) (-136.7392, 9.5101) (-136.8014, 9.5228) (-136.8639, 9.5344) (-136.9266, 9.5455) (-136.9894, 9.5562) (-137.0524, 9.5665) (-137.1155, 9.5762) (-137.1788, 9.5852) (-137.2423, 9.5934) (-137.306, 9.6008) (-137.37, 9.6074) (-137.4341, 9.6133) (-137.4983, 9.6187) (-137.5627, 9.6235) (-137.6272, 9.628) (-137.6918, 9.6319) (-137.7565, 9.6354) (-137.8213, 9.6384) (-137.8862, 9.6408) (-137.9513, 9.6427) (-138.0164, 9.6441) (-138.0817, 9.6451) (-138.1471, 9.6456) (-138.2125, 9.6456) (-138.2781, 9.6453) (-138.3437, 9.6445) (-138.4094, 9.6432) (-138.4752, 9.6416) (-138.541, 9.6395) (-138.607, 9.6371) (-138.673, 9.6342) (-138.739, 9.6309) (-138.8052, 9.6272) (-138.8714, 9.6231) (-138.9377, 9.6186) (-139.004, 9.6137) (-139.0704, 9.6085) (-139.1369, 9.6029) (-139.2034, 9.5969) (-139.27, 9.5905) (-139.3366, 9.5838) (-139.4032, 9.5767) (-139.47, 9.5692) (-139.5367, 9.5614) (-139.6035, 9.5532) (-139.6704, 9.5447) (-139.7373, 9.5358) (-139.8042, 9.5266) (-139.8712, 9.517) (-139.9382, 9.5071) (-140.0052, 9.4969) (-140.0723, 9.4863) (-140.1394, 9.4753) (-140.2066, 9.4641) (-140.2738, 9.4525) (-140.341, 9.4406) (-140.4082, 9.4283) (-140.4755, 9.4157) (-140.5427, 9.4028) (-140.61, 9.3896) (-140.6774, 9.376) (-140.7447, 9.3622) (-140.8121, 9.348) (-140.8795, 9.3335) (-140.9469, 9.3187) (-141.0143, 9.3036) (-141.0683, 9.2912) (-141.1088, 9.2818) (-141.1357, 9.2755) (-141.1492, 9.2723) knots 0 0 0 0 0 0 0.01428571 0.02857143 0.04285714 0.05714286 0.07142857 0.08571429 0.1 0.11428571 0.12857143 0.14285714 0.15714286 0.17142857 0.18571429 0.2 0.21428571 0.22857143 0.24285714 0.25714286 0.27142857 0.28571429 0.3 0.31428571 0.32857143 0.34285714 0.35714286 0.37142857 0.38571429 0.4 0.41428571 0.42857143 0.44285714 0.45714286 0.47142857 0.48571429 0.5 0.51428571 0.52857143 0.54285714 0.55714286 0.57142857 0.58571429 0.6 0.61428571 0.62857143 0.64285714 0.65714286 0.67142857 0.68571429 0.7 0.71428571 0.72857143 0.74285714 0.75714286 0.77142857 0.78571429 0.8 0.81428571 0.82857143 0.84285714 0.85714286 0.87142857 0.88571429 0.9 0.91428571 0.92857143 0.94285714 0.95714286 0.97142857 0.98571429 1 1 1 1 1 1
  arc A94 (-141.1492, 9.2723) -> (-141.6122, 7.5446) centre (-110, 0) ccw
  spline S47 degree 5 poles (-141.6122, 7.5446) (-141.6021, 7.5351) (-141.5819, 7.5161) (-141.5515, 7.4877) (-141.511, 7.45) (-141.4601, 7.4032) (-141.4092, 7.3567) (-141.3581, 7.3104) (-141.3068, 7.2645) (-141.2554, 7.2188) (-141.2039, 7.1734) (-141.1522, 7.1283) (-141.1004, 7.0835) (-141.0484, 7.0389) (-140.9963, 6.9947) (-140.9441, 6.9508) (-140.8917, 6.9072) (-140.8392, 6.8638) (-140.7865, 6.8208) (-140.7337, 6.7781) (-140.6808, 6.7357) (-140.6277, 6.6936) (-140.5745, 6.6518) (-140.5212, 6.6104) (-140.4677, 6.5692) (-140.414, 6.5284) (-140.3603, 6.4879) (-140.3063, 6.4478) (-140.2523, 6.408) (-140.1981, 6.3685) (-140.1438, 6.3293) (-140.0893, 6.2906) (-140.0347, 6.2521) (-139.98, 6.214) (-139.9251, 6.1763) (-139.8701, 6.1389) (-139.8149, 6.1019) (-139.7596, 6.0652) (-139.7042, 6.029) (-139.6486, 5.9931) (-139.5929, 5.9575) (-139.537, 5.9224) (-139.481, 5.8877) (-139.4249, 5.8534) (-139.3686, 5.8195) (-139.3121, 5.786) (-139.2556, 5.7529) (-139.1989, 5.7202) (-139.142, 5.688) (-139.085, 5.6561) (-139.0279, 5.6248) (-138.9706, 5.5939) (-138.9131, 5.5636) (-138.8555, 5.5337) (-138.7977, 5.5044) (-138.7398, 5.4755) (-138.6818, 5.4471) (-138.6236, 5.4191) (-138.5653, 5.3917) (-138.5068, 5.3647) (-138.4481, 5.3385) (-138.3892, 5.313) (-138.3301, 5.2883) (-138.2708, 5.2645) (-138.2113, 5.2414) (-138.1516, 5.2188) (-138.0919, 5.1967) (-138.0321, 5.1749) (-137.9721, 5.1537) (-137.9119, 5.1336) (-137.8513, 5.1152) (-137.8023, 5.1025) (-137.7653, 5.0942) (-137.7405, 5.0893) (-137.728, 5.0871) knots -1 -1 -1 -1 -1 -1 -0.98571429 -0.97142857 -0.95714286 -0.94285714 -0.92857143 -0.91428571 -0.9 -0.88571429 -0.87142857 -0.85714286 -0.84285714 -0.82857143 -0.81428571 -0.8 -0.78571429 -0.77142857 -0.75714286 -0.74285714 -0.72857143 -0.71428571 -0.7 -0.68571429 -0.67142857 -0.65714286 -0.64285714 -0.62857143 -0.61428571 -0.6 -0.58571429 -0.57142857 -0.55714286 -0.54285714 -0.52857143 -0.51428571 -0.5 -0.48571429 -0.47142857 -0.45714286 -0.44285714 -0.42857143 -0.41428571 -0.4 -0.38571429 -0.37142857 -0.35714286 -0.34285714 -0.32857143 -0.31428571 -0.3 -0.28571429 -0.27142857 -0.25714286 -0.24285714 -0.22857143 -0.21428571 -0.2 -0.18571429 -0.17142857 -0.15714286 -0.14285714 -0.12857143 -0.11428571 -0.1 -0.08571429 -0.07142857 -0.05714286 -0.04285714 -0.02857143 -0.01428571 0 0 0 0 0 0
  line L47 (-137.728, 5.0871) -> (-137.6286, 5.0688)
  arc A95 (-136.8197, 3.9399) -> (-137.6286, 5.0688) centre (-137.809, 4.0852) ccw
  circle A96 centre (-110, 0) radius 2.25
  circle A97 centre (0, 23) radius 2.3
  circle A98 centre (-110, 23) radius 2.3
  dimension "d54" = 4.6
  dimension "d55" = 23
  dimension "d56" = 4.6
  measures "d54" diameter of A97
  measures "d55" distance of origin A97.centre
  measures "d56" diameter of A98
extrude "Extrude15" cut sketch "Sketch21" against normal blind 3.3 contours A98 bodies 3
extrude "Extrude16" cut sketch "Sketch21" against normal blind 3.3 contours A97 bodies 2
named bodies: "gear1", "gear2", "gear3"
